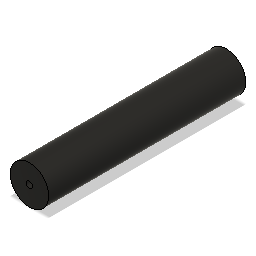
Rol v6 (Autodesk Fusion 360 design; units mm, degrees)
Autodesk Fusion 360 part; units mm, degrees
sketch "Sketch1" plane through (0, 0, 0) normal (0, 0, 1) x (1, 0, 0)
  circle A0 centre (0, 0) radius 4.1
  circle A1 centre (0, 0) radius 25
  dimension "d1" = 8.2
  dimension "d2" = 50
  constraint coincident A0.centre A1.centre
  constraint concentric A0 A1
  measures "d1" diameter of A0
  measures "d2" diameter of A1
extrude "Extrude1" add sketch "Sketch1" along normal blind 256
